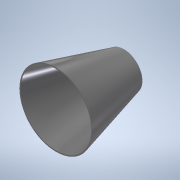
# Autodesk Inventor part: Redukcja symetryczna Ø101,6x51x1,6 L=94,7
Saved by Autodesk Inventor 2020 (Build 240168000, 168)
## iProperties
RuleStatus: InUse
Created: 2022-03-21
Part Number: Redukcja symetryczna Ø101,6x51x1,6 L=94,7
Material: 304
Description: Redukcja symetryczna Ø101,6x51x1,6 L=94,7
Document SubType Name: Modelowanie
Designer: Radosław
Density: 8 g/cm^3
Sheet Metal Rule: 1,5
Sheet Metal Width: 0,000 mm
Sheet Metal Length: 0,000 mm
Sheet Metal Area: 0,000 mm^2
Appearance: Częściowo polerowany(1)
Author: Radosław
Autodesk Inventor part; units mm, degrees
ref_plane "YZ Plane" through (0, 0, 0) normal (1, 0, 0) x (0, 1, 0)
ref_plane "XY Plane" through (0, 0, 0) normal (0, 0, 1) x (1, 0, 0)
sketch "Szkic6" plane through (0, 0, 0) normal (0, 1, 0) x (-1, 0, 0)
  circle A0 centre (0, 0) radius 50.8
  dimension "d33" = 101.6
  constraints: 1 centre point, 1 coincident
  measures "d33" diameter of A0
ref_plane "Płaszczyzna konstrukcyjna1" through (0, 94.7, 0) normal (0, 1, 0) x (-1, 0, 0)
sketch "Szkic7" plane through (0, 94.7, 0) normal (0, 1, 0) x (-1, 0, 0)
  circle A0 centre (0, 0) radius 25.5
  dimension "d35" = 51
  constraints: 1 centre point, 1 coincident
  measures "d35" diameter of A0
loft "Wyciągnięcie złożone1" add profiles "Szkic6", "Szkic7"
shell "Skorupa1" thickness 1.6 removed faces 2 at (4.5479, 94.7, -4.6843) at (7.3018, 0, 11.5135)
equation "\"d33\" = OD1"
equation "\"d35\" = OD2"
equation "\"d52\" = THK"
equation "\"SzerokośćGięciaPodcięcia\" = Grubość"
equation "\"RozmiarPodcięciaNarożnika\" = 4 * Grubość"
equation "\"PromieńPrzejścia\" = PromieńGięcia"
equation "\"Rozmiar_promienia_Jacobiego\" = PromieńGięcia"
equation "\"Wielk_odstępu\" = Grubość"
equation "\"d2\" = PromieńGięcia"
equation "\"d23\" = PromieńGięcia"
equation "\"OD1\" = 101.6"
equation "\"OD2\" = 51"
equation "\"L\" = 94.7"
equation "\"THK\" = 1.6"
equation "\"d34\" = L"
equation "\"Grubość\" = 1.5"
equation "\"PromieńGięcia\" = 3"
